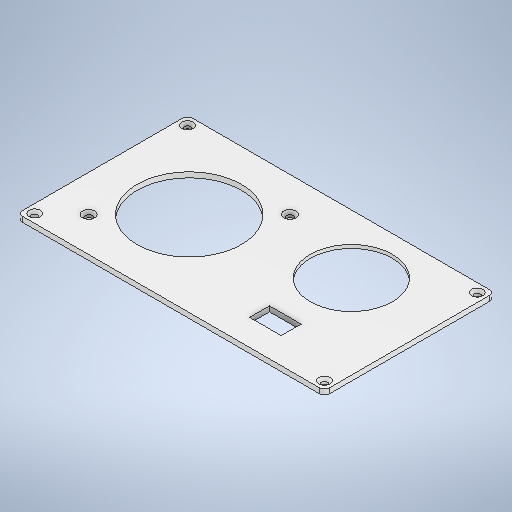
# Autodesk Inventor part: 4.L - GM - 01.02
Saved by Autodesk Inventor 2025.2 (Build 292293000, 293)
## iProperties
Created: 2025-03-02
Part Number: 4.L - GM - 01.02
Material: LCP plast
Document SubType Name: Modeling
Designer: hepma_axt67em
Density: 1.626 g/cm^3
Appearance: Hladká – bílá
Author: HEP
Autodesk Inventor part; units mm, degrees
ref_plane "YZ Plane" through (0, 0, 0) normal (1, 0, 0) x (0, 1, 0)
ref_plane "XZ Plane" through (0, 0, 0) normal (0, 1, 0) x (-1, 0, 0)
ref_plane "XY Plane" through (0, 0, 0) normal (0, 0, 1) x (1, 0, 0)
sketch "Náčrt1" plane through (0, 0, 0) normal (0, 1, 0) x (-1, 0, 0)
  line L0 (0, -68.6) -> (0, 68.6) projected
  line L1 (-123.9, 0) -> (123.9, 0) projected
  line L2 (88.5, -49) -> (-88.5, -49)
  line L3 (-88.5, -49) -> (-88.5, 49)
  line L4 (-88.5, 49) -> (88.5, 49)
  line L5 (88.5, 49) -> (88.5, -49)
  point P0 (0, 0)
  dimension "d0" = 177
  dimension "d1" = 98
  constraints: 8 end point, 2 parallel, 1 horizontal, 1 perpendicular, 2 other
  measures "d0" distance of L2.start L2.end
  measures "d1" distance of L2.end L3.end
extrude "Vysunutí1" add sketch "Náčrt1" along normal blind 3
sketch "Náčrt2" plane through (0, 3, 0) normal (0, 1, 0) x (1, 0, 0)
  line L0 (0, 68.6) -> (0, -68.6) projected
  line L1 (123.9, 0) -> (-123.9, 0) projected
  point P0 (0, 0)
  point P1 (-83.55, 44.05)
  point P2 (-83.55, -44.05)
  point P3 (83.55, -44.05)
  point P4 (83.55, 44.05)
  dimension "d4" = 88.1
  dimension "d5" = 167.1
  dimension "d6" = 88.1
  dimension "d7" = 167.1
  constraints: 2 symmetric about line
  measures "d4" distance of point (-83.55, -44.05) point (-83.55, 44.05)
  measures "d5" distance of point (-83.55, -44.05) point (83.55, -44.05)
  measures "d6" distance of point (83.55, 44.05) point (83.55, -44.05)
  measures "d7" distance of point (-83.55, 44.05) point (83.55, 44.05)
hole "Díra1" at (-83.55, 3, -44.05) at (-83.55, 3, 44.05) at (83.55, 3, 44.05) at (83.55, 3, -44.05) direction (0, -1, 0) diameter 3.4 end through all clearance for "Šroub se zápustnou hlavou ISO 2009/7046" size "M3" standard "ISO"
fillet "Zaoblení1" radius 3 4 edges at (88.5, 1.5, 49) (88.5, 1.5, -49) (-88.5, 1.5, 49) (-88.5, 1.5, -49)
sketch "Náčrt3" plane through (0, 3, 0) normal (0, 1, 0) x (1, 0, 0)
  line L0 (123.9, 0) -> (-123.9, 0) projected
  line L1 (-88.5, 46) -> (-88.5, -46) projected
  point P0 (0, 0)
  point P1 (-38.5, 0)
  dimension "d21" = 50
  constraints: 1 point on line
  measures "d21" distance from line of L1 point (-38.5, 0)
hole "Díra2" at (-38.5, 3, 0) direction (0, -1, 0) diameter 60.1 end through all
sketch "Náčrt4" plane through (0, 0, 0) normal (0, -1, 0) x (1, 0, 0)
  line L0 (0, 68.6) -> (0, -68.6) projected
  line L1 (-123.9, 0) -> (123.9, 0) projected
  point P0 (0, 0)
  point P1 (40, -15)
  dimension "d29" = 40
  dimension "d38" = 15
  measures "d29" distance from line of L0 point (40, -15)
  measures "d38" distance from line of L1 point (40, -15)
hole "Díra3" at (40, 0, -15) direction (0, 1, 0) diameter 47.3 end through all counterbore diameter 50.3 counterbore depth 1
sketch "Náčrt5" plane through (0, 3, 0) normal (0, 1, 0) x (1, 0, 0)
  line L0 (30.3, -22.5) -> (48.5, -22.5)
  line L1 (48.5, -22.5) -> (48.5, -34)
  line L2 (48.5, -34) -> (30.3, -34)
  line L3 (30.3, -34) -> (30.3, -22.5)
  line L4 (-85.5, -49) -> (85.5, -49) projected
  line L5 (88.5, -46) -> (88.5, 46) projected
  point P0 (0, 0)
  dimension "d39" = 18.2
  dimension "d40" = 11.5
  dimension "d41" = 15
  dimension "d43" = 40
  constraints: 8 end point, 2 parallel, 1 horizontal, 1 perpendicular
  measures "d39" distance of L1.end L2.end
  measures "d40" distance of L0.end L1.end
  measures "d41" distance between parallel lines of L4 L2
  measures "d43" distance between parallel lines of L5 L1
extrude "Vysunutí2" cut sketch "Náčrt5" against normal up to surface (3 mm away)
sketch "Náčrt6" plane through (0, 3, 0) normal (0, 1, 0) x (1, 0, 0)
  line L0 (123.9, 0) -> (-123.9, 0) projected
  line L1 (0, 68.6) -> (0, -68.6) projected
  circle A0 centre (-38.5, 0) radius 30.05 projected
  point P0 (0, 0)
  point P1 (-67.5, -29)
  point P2 (-9.5, 29)
  dimension "d46" = 29
  dimension "d49" = 29
  dimension "d57" = 29
  dimension "d58" = 29
  measures "d46" horizontal distance of A0.centre point (-67.5, -29)
  measures "d49" horizontal distance of A0.centre point (-9.5, 29)
  measures "d57" distance from line of L0 point (-9.5, 29)
  measures "d58" distance from line of L0 point (-67.5, -29)
hole "Díra4" at (-67.5, 3, 29) at (-9.5, 3, -29) direction (0, -1, 0) diameter 3.9 end through all
chamfer "Zkosení1" distance 1.5 angle 45 6 edges at (-83.55, 3, 42.35) (-83.55, 3, -45.75) (83.55, 3, -45.75) (83.55, 3, 42.35) (-67.5, 3, 27.05) (-9.5, 3, -30.95)
